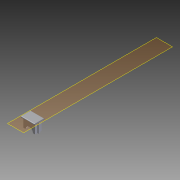
# Autodesk Inventor part: InternalKey
Saved by Autodesk Inventor 2012 (Build 160160000, 160)
## iProperties
Created: 2011-09-20
Part Number: InternalKey
Material: Default
Document SubType Name: Modeling
Designer: KuttaA
Density: 1 g/cm^3
Mass: 2.21175 g
Surface Area: 14.0837 cm^2
Volume: 2.21175 cm^3
Author: KuttaA
Autodesk Inventor part; units mm, degrees
ref_plane "YZ Plane" through (0, 0, 0) normal (1, 0, 0) x (0, 1, 0)
ref_plane "XZ Plane" through (0, 0, 0) normal (0, 1, 0) x (-1, 0, 0)
ref_plane "XY Plane" through (0, 0, 0) normal (0, 0, 1) x (1, 0, 0)
ref_plane "Work Plane8" through (7.15, 0.8, 25.4) normal (0, 1, 0) x (1, 0, 0)
sketch "Sketch21" plane through (7.15, 0.8, 25.4) normal (0, 1, 0) x (1, 0, 0)
  line L0 (-3, 3) -> (-24, 3) projected
  line L1 (-3, 197) -> (-3, 3) projected
  line L2 (-24, 197) -> (-3, 197) projected
  line L3 (-24, 3) -> (-24, 197) projected
  line L4 (-4.82, 19.3667) -> (-3.32, 19.3667) projected
  line L5 (-3.32, 19.3667) -> (-3.32, 16.0333) projected
  line L6 (-3.32, 16.0333) -> (-4.82, 16.0333) projected
  line L7 (-4.82, 16.0333) -> (-4.82, 12.7) projected
  line L8 (-4.82, 12.7) -> (-22.18, 12.7) projected
  line L9 (-22.18, 12.7) -> (-22.18, 16.0333) projected
  line L10 (-22.18, 16.0333) -> (-23.68, 16.0333) projected
  line L11 (-23.68, 16.0333) -> (-23.68, 19.3667) projected
  line L12 (-23.68, 19.3667) -> (-22.18, 19.3667) projected
  line L13 (-22.18, 19.3667) -> (-22.18, 22.7) projected
  line L14 (-22.18, 22.7) -> (-4.82, 22.7) projected
  line L15 (-4.82, 22.7) -> (-4.82, 19.3667) projected
  line L16 (-21.88, 22.4) -> (-21.88, 19.0667)
  line L17 (-21.88, 19.0667) -> (-23.38, 19.0667)
  line L18 (-23.38, 19.0667) -> (-23.38, 16.3333)
  line L19 (-23.38, 16.3333) -> (-21.88, 16.3333)
  line L20 (-21.88, 16.3333) -> (-21.88, 13)
  line L21 (-21.88, 13) -> (-5.12, 13)
  line L22 (-5.12, 13) -> (-5.12, 16.3333)
  line L23 (-5.12, 16.3333) -> (-3.62, 16.3333)
  line L24 (-3.62, 16.3333) -> (-3.62, 19.0667)
  line L25 (-3.62, 19.0667) -> (-5.12, 19.0667)
  line L26 (-5.12, 19.0667) -> (-5.12, 22.4)
  line L27 (-5.12, 22.4) -> (-21.88, 22.4)
  point P0 (-7.15, 25.4)
  dimension "d99" = 0.3
  dimension "d100" = 0.3
  dimension "d101" = 0.3
  dimension "d102" = 0.3
  dimension "d103" = 0.3
  dimension "d104" = 0.3
  dimension "d105" = 0.3
  dimension "d106" = 0.3
  dimension "d107" = 0.3
  dimension "d108" = 0.3
  dimension "d109" = 0.3
  dimension "d110" = 0.3
  constraints: 24 end point, 8 parallel, 2 collinear, 2 perpendicular
  measures "d99" distance between parallel lines of L14 L27
  measures "d100" distance between parallel lines of L15 L26
  measures "d101" distance between parallel lines of L4 L25
  measures "d102" distance between parallel lines of L5 L24
  measures "d103" distance between parallel lines of L6 L23
  measures "d104" distance between parallel lines of L7 L22
  measures "d105" distance between parallel lines of L8 L21
  measures "d106" distance between parallel lines of L9 L20
  measures "d107" distance between parallel lines of L10 L19
  measures "d108" distance between parallel lines of L11 L18
  measures "d109" distance between parallel lines of L12 L17
  measures "d110" distance between parallel lines of L13 L16
ref_plane "Work Plane9" through (-1.05, -12.7, 2.7) normal (0, 1, 0) x (0, 0, 1)
extrude "Extrusion20" add sketch "Sketch21" against normal up to surface (13.5 mm away) contours L27 L26 L25 L24 L23 L22 L21 L20 L19 L18 L17 L16
sketch "Sketch22" plane through (-14.73, 0.8, 12.4) normal (0, 0, 1) x (1, 0, 0)
  circle A0 centre (8.38, -13.5) radius 5 construction
  arc A1 (3.08, -13.5) -> (13.68, -13.5) centre (8.38, -13.5) ccw projected
  arc A2 (13.68, -13.5) -> (3.08, -13.5) centre (8.38, -13.5) ccw
  point P0 (14.73, -0.8)
  constraints: 2 point on circle, 1 centre point, 1 concentric
extrude "Extrusion21" cut sketch "Sketch22" against normal through all
sketch "Sketch23" plane through (7.15, 0.8, 25.4) normal (0, 1, 0) x (1, 0, 0)
  line L0 (-21.88, 22.4) -> (-21.88, 19.0667) projected
  line L1 (-21.88, 19.0667) -> (-23.38, 19.0667) projected
  line L2 (-23.38, 19.0667) -> (-23.38, 16.3333) projected
  line L3 (-23.38, 16.3333) -> (-21.88, 16.3333) projected
  line L4 (-21.88, 16.3333) -> (-21.88, 13) projected
  line L5 (-21.88, 13) -> (-5.12, 13) projected
  line L6 (-5.12, 13) -> (-5.12, 16.3333) projected
  line L7 (-5.12, 16.3333) -> (-3.62, 16.3333) projected
  line L8 (-3.62, 16.3333) -> (-3.62, 19.0667) projected
  line L9 (-3.62, 19.0667) -> (-5.12, 19.0667) projected
  line L10 (-5.12, 19.0667) -> (-5.12, 22.4) projected
  line L11 (-5.12, 22.4) -> (-21.88, 22.4) projected
  line L12 (-24, 3) -> (-24, 197) projected
  line L13 (-3, 197) -> (-3, 3) projected
  line L14 (-23.68, 24.9) -> (-3.32, 24.9)
  line L15 (-3.32, 24.9) -> (-3.32, 10.5)
  line L16 (-3.32, 10.5) -> (-23.68, 10.5)
  line L17 (-23.68, 10.5) -> (-23.68, 24.9)
  point P0 (-7.15, 25.4)
  dimension "d115" = 2.5
  dimension "d116" = 2.5
  dimension "d117" = 0.3
  dimension "d118" = 0.3
  constraints: 8 end point, 2 parallel, 1 horizontal, 1 perpendicular
  measures "d115" distance between parallel lines of L14 L11
  measures "d116" distance between parallel lines of L16 L5
  measures "d117" distance between parallel lines of L2 L17
  measures "d118" distance between parallel lines of L15 L8
extrude "Extrusion22" add sketch "Sketch23" along normal blind 1.5 contours L11 L10 L9 L8 L7 L6 L5 L4 L3 L2 L1 L0 | L14 L15 L16 L17
sketch "Sketch24" plane through (-16.53, 0.8, 14.9) normal (0, 0, 1) x (1, 0, 0)
  line L0 (20.36, 1.5) -> (0, 1.5) projected
  line L1 (0, 0) -> (0, 1.5) projected
  line L2 (20.36, 0) -> (0, 0) projected
  line L3 (20.36, 0) -> (20.36, 1.5) projected
  line L4 (6.7867, 0) -> (13.5733, 0)
  line L5 (13.5733, 0) -> (13.5733, 0.75)
  line L6 (13.5733, 0.75) -> (6.7867, 0.75)
  line L7 (6.7867, 0.75) -> (6.7867, 0)
  point P0 (16.53, -0.8)
  dimension "d121" = 20.36
  dimension "d122" = 6.7867
  dimension "d123" = 6.7867
  dimension "d124" = 0.75
  dimension "d125" = 1.5
  constraints: 8 end point, 2 parallel, 1 horizontal, 1 perpendicular, 1 point on line
  measures "d121" distance of L2.start L1.start
  measures "d122" distance of L5.end L6.end
  measures "d123" distance between parallel lines of L3 L5
  measures "d124" distance between parallel lines of L2 L6
  measures "d125" distance between parallel lines of L2 L0
extrude "Extrusion23" cut sketch "Sketch24" against normal blind 1.5 contours L2 L7 L6 L5
sketch "Sketch25" plane through (3.83, 0.8, 0.5) normal (0, 0, -1) x (-1, 0, 0)
  line L0 (6.7867, 0.75) -> (6.7867, 0) projected
  line L1 (13.5733, 0.75) -> (6.7867, 0.75) projected
  line L2 (13.5733, 0) -> (13.5733, 0.75) projected
  line L3 (20.36, 0) -> (0, 0) projected
  point P0 (3.83, -0.8)
fillet "Fillet13" radius 2 3 edges at (-9.7433, 1.55, 14.15) (-2.9567, 1.55, 14.15) (-6.35, 1.55, 13.4)
extrude "Extrusion24" cut sketch "Sketch25" against normal blind 1.5
fillet "Fillet14" radius 2 3 edges at (-2.9567, 1.55, 1.25) (-9.7433, 1.55, 1.25) (-6.35, 1.55, 2)
fillet "Fillet15" radius 1 8 edges at (-6.35, 2.3, 0.5) (3.83, 2.3, 7.7) (-6.35, 2.3, 14.9) (-16.53, 2.3, 7.7) (3.83, 1.55, 0.5) (3.83, 1.55, 14.9) (-16.53, 1.55, 0.5) (-16.53, 1.55, 14.9)
sketch "Sketch26" plane through (-16.23, -12.7, 9.0667) normal (0, -1, 0) x (1, 0, 0)
  line L0 (4.58, -6.0667) -> (4.58, 3.3333) projected
  line L1 (4.58, 3.3333) -> (1.5, 3.3333) projected
  line L2 (1.5, 3.3333) -> (1.5, 0) projected
  line L3 (1.5, 0) -> (0, 0) projected
  line L4 (0, 0) -> (0, -2.7333) projected
  line L5 (0, -2.7333) -> (1.5, -2.7333) projected
  line L6 (1.5, -2.7333) -> (1.5, -6.0667) projected
  line L7 (1.5, -6.0667) -> (4.58, -6.0667) projected
  line L8 (15.18, 3.3333) -> (15.18, -6.0667) projected
  line L9 (15.18, -6.0667) -> (18.26, -6.0667) projected
  line L10 (18.26, -6.0667) -> (18.26, -2.7333) projected
  line L11 (18.26, -2.7333) -> (19.76, -2.7333) projected
  line L12 (19.76, -2.7333) -> (19.76, 0) projected
  line L13 (19.76, 0) -> (18.26, 0) projected
  line L14 (18.26, 0) -> (18.26, 3.3333) projected
  line L15 (18.26, 3.3333) -> (15.18, 3.3333) projected
  point P0 (16.23, -9.0667)
extrude "Extrusion25" cut sketch "Sketch26" against normal blind 0.15
sketch "Sketch27" plane through (7.15, 0.8, 25.4) normal (0, -1, 0) x (1, 0, 0)
  line L0 (-3.62, -16.3333) -> (-3.62, -19.0667) projected
  line L1 (-3.62, -19.0667) -> (-5.12, -19.0667) projected
  line L2 (-5.12, -19.0667) -> (-5.12, -22.4) projected
  line L3 (-5.12, -22.4) -> (-21.88, -22.4) projected
  line L4 (-21.88, -22.4) -> (-21.88, -19.0667) projected
  line L5 (-21.88, -19.0667) -> (-23.38, -19.0667) projected
  line L6 (-23.38, -19.0667) -> (-23.38, -16.3333) projected
  line L7 (-23.38, -16.3333) -> (-21.88, -16.3333) projected
  line L8 (-21.88, -16.3333) -> (-21.88, -13) projected
  line L9 (-21.88, -13) -> (-5.12, -13) projected
  line L10 (-5.12, -13) -> (-5.12, -16.3333) projected
  line L11 (-5.12, -16.3333) -> (-3.62, -16.3333) projected
  arc A0 (-22.68, -10.5) -> (-23.68, -11.5) centre (-22.68, -11.5) ccw projected
  line L12 (-23.68, -11.5) -> (-23.68, -23.9) projected
  arc A1 (-23.68, -23.9) -> (-22.68, -24.9) centre (-22.68, -23.9) ccw projected
  line L13 (-22.68, -24.9) -> (-16.8933, -24.9) projected
  line L14 (-16.8933, -24.9) -> (-16.8933, -23.4) projected
  line L15 (-16.8933, -23.4) -> (-10.1067, -23.4) projected
  line L16 (-10.1067, -23.4) -> (-10.1067, -24.9) projected
  line L17 (-10.1067, -24.9) -> (-4.32, -24.9) projected
  arc A2 (-4.32, -24.9) -> (-3.32, -23.9) centre (-4.32, -23.9) ccw projected
  line L18 (-3.32, -23.9) -> (-3.32, -11.5) projected
  arc A3 (-3.32, -11.5) -> (-4.32, -10.5) centre (-4.32, -11.5) ccw projected
  line L19 (-4.32, -10.5) -> (-10.1067, -10.5) projected
  line L20 (-10.1067, -10.5) -> (-10.1067, -12) projected
  line L21 (-10.1067, -12) -> (-16.8933, -12) projected
  line L22 (-16.8933, -12) -> (-16.8933, -10.5) projected
  line L23 (-16.8933, -10.5) -> (-22.68, -10.5) projected
  point P0 (-7.15, -25.4)
extrude "Extrusion26" cut sketch "Sketch27" against normal blind 0.15
equation "\"d100\" = d99"
equation "\"d101\" = d99"
equation "\"d102\" = d101"
equation "\"d103\" = d102"
equation "\"d104\" = d102"
equation "\"d105\" = d104"
equation "\"d106\" = d105"
equation "\"d107\" = d106"
equation "\"d108\" = d106"
equation "\"d109\" = d107"
equation "\"d110\" = d109"
equation "\"d116\" = d115"
equation "\"d118\" = d117"
equation "\"d122\" = 0.333333 * d121"
equation "\"d123\" = d122"
equation "\"d124\" = 0.5 * d125"
body "Solid5"
